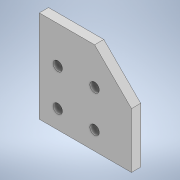
# Autodesk Inventor part: 2.5x2.5
Saved by Autodesk Inventor 2020 (Build 240168000, 168)
## iProperties
Created: 2020-01-14
Part Number: 2.5x2.5
Material: Generic
Document SubType Name: Modeling
Designer: 339294
Density: 1 g/cm^3
Appearance: Default
Author: 339294
Autodesk Inventor part; units mm, degrees
ref_plane "YZ Plane" through (0, 0, 0) normal (1, 0, 0) x (0, 1, 0)
ref_plane "XZ Plane" through (0, 0, 0) normal (0, 1, 0) x (-1, 0, 0)
ref_plane "XY Plane" through (0, 0, 0) normal (0, 0, 1) x (1, 0, 0)
sketch "Sketch1" plane through (0, 0, 0) normal (0, 0, 1) x (1, 0, 0)
  line L0 (0, 0) -> (50.8, 0)
  line L1 (38.1, 63.5) -> (0, 63.5)
  line L2 (0, 63.5) -> (0, 0)
  line L3 (50.8, 0) -> (63.5, 0)
  line L4 (63.5, 0) -> (63.5, 38.1)
  line L5 (38.1, 63.5) -> (63.5, 38.1)
  circle A0 centre (12.7, 12.7) radius 3.2512
  circle A1 centre (12.7, 38.1) radius 3.2512
  circle A2 centre (38.1, 12.7) radius 3.2512
  circle A3 centre (38.1, 38.1) radius 3.2512
  dimension "d10" = 63.5
  dimension "d11" = 50.8
  dimension "d12" = 38.1
  dimension "d14" = 38.1
  dimension "d15" = 25.4
  dimension "d16" = 25.4
  dimension "d17" = 6.5024
  dimension "d18" = 12.7
  dimension "d19" = 12.7
  dimension "d22" = 25.4
  dimension "d25" = 25.4
  constraints: 12 end point, 4 centre point, 3 horizontal, 1 parallel, 1 perpendicular, 1 vertical, 6 other
  measures "d10" distance of L1.end L0.start
  measures "d11" distance of L0.start L0.end
  measures "d12" distance of L3.end L4.end
  measures "d14" distance of L1.start L1.end
  measures "d15" horizontal distance of L1.start L4.end
  measures "d16" horizontal distance of L1.start L4.end
  measures "d17" diameter of A0
  measures "d18" distance from line of L0 A0.centre
  measures "d19" distance from line of L2 A0.centre
  measures "d22" distance of A0.centre A1.centre
  measures "d25" distance of A0.centre A2.centre
extrude "Extrusion1" add sketch "Sketch1" along normal blind 6.35
body "Solid1"
